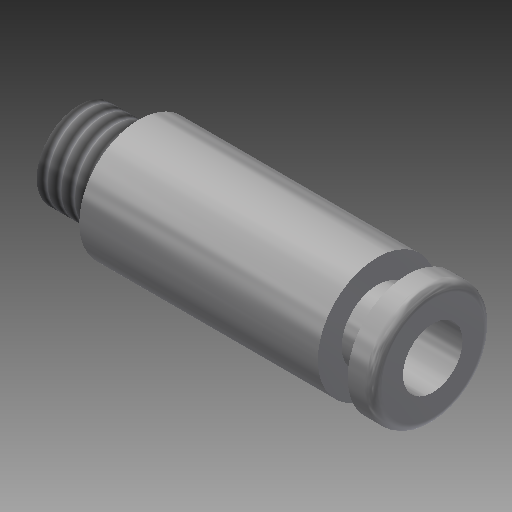
# Autodesk Inventor part: Schlauchfitting
Saved by Autodesk Inventor 2018 (Build 220112000, 112)
## iProperties
Created: 2011-11-24
Part Number: Schlauchfitting
Material: Stainless Steel
Document SubType Name: Modeling
Designer: Neef
Mass: 4.31131 g
Surface Area: 7.25684 cm^2
Volume: 0.538913 cm^3
Density: 8 g/cm^3
Appearance: Steel
Author: Neef
Autodesk Inventor part; units mm, degrees
ref_plane "YZ Plane" through (0, 0, 0) normal (1, 0, 0) x (0, 1, 0)
ref_plane "XZ Plane" through (0, 0, 0) normal (0, 1, 0) x (-1, 0, 0)
ref_plane "XY Plane" through (0, 0, 0) normal (0, 0, 1) x (1, 0, 0)
sketch "Skizze1" plane through (0, 0, 0) normal (0, 0, 1) x (1, 0, 0)
  line L0 (0, 4) -> (0, 0.5) projected
  line L1 (-4.15, 0) -> (24.9, 0) projected
  line L2 (0, 2.5) -> (3.5, 2.5)
  line L3 (3.5, 2.5) -> (3.5, 3.5)
  line L4 (3.5, 3.5) -> (17.5, 3.5)
  line L5 (17.5, 3.5) -> (17.5, 2.1)
  line L6 (17.5, 2.1) -> (19.25, 2.1)
  line L7 (19.25, 2.1) -> (19.25, 3.5)
  line L8 (19.25, 3.5) -> (20.75, 3.5)
  line L9 (20.75, 3.5) -> (20.75, 1.75)
  line L10 (7.75, 1) -> (0, 1)
  line L11 (0, 1) -> (0, 2.5)
  line L12 (20.75, 1.75) -> (7.75, 1.75)
  line L13 (7.75, 1.75) -> (7.75, 1)
  dimension "d0" = 1
  dimension "d1" = 3.5
  dimension "d2" = 2.5
  dimension "d3" = 2.1
  dimension "d4" = 1.5
  dimension "d5" = 1.75
  dimension "d6" = 14
  dimension "d7" = 3.5
  dimension "d11" = 1.75
  dimension "d12" = 13
  constraints: 24 end point, 7 parallel, 5 perpendicular, 2 point on line, 1 collinear
  measures "d0" distance between parallel lines of L1 L10
  measures "d1" distance between parallel lines of L1 L4
  measures "d2" distance between parallel lines of L1 L2
  measures "d3" distance between parallel lines of L1 L6
  measures "d4" distance of L7.end L8.end
  measures "d5" distance of L5.end L6.end
  measures "d6" distance of L3.end L4.end
  measures "d7" distance of L2.start L2.end
  measures "d11" distance between parallel lines of L1 L12
  measures "d12" distance of L9.end L12.end
revolve "Umdrehung1" add sketch "Skizze1" angle 360 about axis through (0, 0, 0) along (1, 0, 0)
thread "Gewinde1" size "M5x0.8" class "6g" standard "ANSI Metric M Profile" full length
fillet "Rundung1" radius 0.5 1 edges at (20.75, -3.5, 0)
